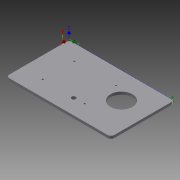
# Autodesk Inventor part: capac 2
Saved by Autodesk Inventor 2015 SP1 (Build 190203100, 203)
## iProperties
Created: 2015-04-26
Part Number: capac 2
Material: Generic
Document SubType Name: Modeling
Designer: ubik
Density: 1 g/cm^3
Appearance: Default
Author: ubik
Autodesk Inventor part; units mm, degrees
ref_plane "YZ Plane" through (0, 0, 0) normal (1, 0, 0) x (0, 1, 0)
ref_plane "XZ Plane" through (0, 0, 0) normal (0, 1, 0) x (-1, 0, 0)
ref_plane "XY Plane" through (0, 0, 0) normal (0, 0, 1) x (1, 0, 0)
sketch "Sketch1" plane through (0, 0, 0) normal (0, 0, 1) x (1, 0, 0)
  line L0 (0, 0) -> (200, 0)
  line L1 (200, 0) -> (200, 120)
  line L2 (200, 120) -> (0, 120)
  line L3 (0, 120) -> (0, 0)
  dimension "width" = 200
  dimension "height" = 120
  constraints: 8 end point, 2 parallel, 1 horizontal, 1 perpendicular
  measures "width" distance of L1.end L2.end
  measures "height" distance of L2.end L0.start
extrude "Extrusion1" add sketch "Sketch1" along normal blind 5
sketch "Sketch2" plane through (0, 0, 5) normal (0, 0, 1) x (1, 0, 0)
  circle A0 centre (150, 70) radius 37
  line L0 (85, 44) -> (115, 44)
  line L1 (115, 44) -> (115, 14)
  line L2 (115, 14) -> (85, 14)
  line L3 (85, 14) -> (85, 44)
  line L4 (0, 120) -> (0, 0) projected
  line L5 (0, 0) -> (200, 0) projected
  circle A1 centre (100, 29) radius 4
  circle A2 centre (150, 70) radius 21
  dimension "d4" = 74
  dimension "d5" = 30
  dimension "d6" = 30
  dimension "d7" = 85
  dimension "d8" = 70
  dimension "d9" = 150
  dimension "d10" = 8
  dimension "d11" = 42
  constraints: 8 end point, 3 centre point, 2 parallel, 1 coincident, 1 horizontal, 1 perpendicular
  measures "d4" diameter of A0
  measures "d5" distance of L1.end L2.end
  measures "d6" distance of L0.end L1.end
  measures "d7" distance between parallel lines of L4 L3
  measures "d8" distance from line of A0.centre L5
  measures "d9" distance from line of A0.centre L4
  measures "d10" diameter of A1
  measures "d11" diameter of A2
extrude "Extrusion2" cut sketch "Sketch2" against normal blind 8 contours A1 | A2
hole "Hole1" at (40, 90, 5) direction (0, 0, -1) diameter 3 end through all
pattern_linear "Rectangular Pattern1" count 2 spacing 80 along (1, 0, 0) count 2 spacing 60 along (0, -1, 0) of "Hole1"
fillet "Fillet1" radius 6 4 edges at (0, 120, 2.5) (0, 0, 2.5) (200, 0, 2.5) (200, 120, 2.5)
body "Solid1"
